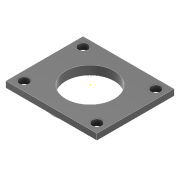
# Autodesk Inventor part: PinholeFlexFixture
Saved by Autodesk Inventor 2022 (Build 260153000, 153)
## iProperties
Created: 2022-02-18
Part Number: PinholeFlexFixture
Material: Acetal Resin, Black
Document SubType Name: Modeling
Designer: eganc
Density: 1.425 g/cm^3
Appearance: Smooth - Black
Author: eganc
Autodesk Inventor part; units mm, degrees
ref_plane "YZ Plane" through (0, 0, 0) normal (1, 0, 0) x (0, 1, 0)
ref_plane "XZ Plane" through (0, 0, 0) normal (0, 1, 0) x (-1, 0, 0)
ref_plane "XY Plane" through (0, 0, 0) normal (0, 0, 1) x (1, 0, 0)
sketch "Sketch1" plane through (0, 0, 0) normal (0, 1, 0) x (-1, 0, 0)
  line L0 (-7.5, 6.36) -> (7.5, 6.36)
  line L1 (7.5, 6.36) -> (7.5, -6.36)
  line L2 (7.5, -6.36) -> (-7.5, -6.36)
  line L3 (-7.5, -6.36) -> (-7.5, 6.36)
  line L4 (-7.5, 6.36) -> (7.5, -6.36) construction
  line L5 (7.5, 6.36) -> (-7.5, -6.36) construction
  point P0 (0, 0)
  dimension "d0" = 12.72
  dimension "d1" = 15
  constraints: 12 end point, 2 midpoint, 2 parallel, 1 horizontal, 1 perpendicular
  measures "d0" distance of L0.end L1.end
  measures "d1" distance of L1.end L2.end
extrude "Extrusion1" add sketch "Sketch1" along normal blind 1
sketch "Sketch2" plane through (0, 1, 0) normal (0, 1, 0) x (1, 0, 0)
  circle A0 centre (0, 0) radius 4
  dimension "d4" = 8
  constraints: 1 centre point, 1 coincident
  measures "d4" diameter of A0
extrude "Extrusion2" cut sketch "Sketch2" against normal up to surface (1 mm away)
sketch "Sketch3" plane through (0, 0, 0) normal (0, -1, 0) x (1, 0, 0)
  circle A0 centre (0, 0) radius 4
  circle A1 centre (0, 0) radius 6
  dimension "d7" = 12
  dimension "d8" = 8
  constraints: 2 centre point, 2 coincident
  measures "d7" diameter of A1
  measures "d8" diameter of A0
extrude "Extrusion3" add sketch "Sketch3" along normal blind 0.46
sketch "Sketch4" plane through (0, 1, 0) normal (0, 1, 0) x (1, 0, 0)
  point P0 (0, 0)
sketch "Sketch5" plane through (0, 1, 0) normal (0, 1, 0) x (1, 0, 0)
  circle A0 centre (-6, -4.86) radius 0.8
  line L0 (-7.5, 6.36) -> (-7.5, -6.36) projected
  line L1 (-7.5, 0) -> (7.5, 0) construction
  line L2 (7.5, -6.36) -> (7.5, 6.36) projected
  line L3 (-7.5, -6.36) -> (7.5, -6.36) projected
  line L4 (0, -6.36) -> (0, 6.36) construction
  line L5 (7.5, 6.36) -> (-7.5, 6.36) projected
  circle A1 centre (-6, 4.86) radius 0.8
  line L6 (0, 6.36) -> (0, -6.36) construction
  circle A2 centre (6, -4.86) radius 0.8
  circle A3 centre (6, 4.86) radius 0.8
  point P0 (0, 0)
  dimension "d11" = 1.5
  dimension "d12" = 1.6
  dimension "d13" = 1.5
  constraints: 6 end point, 5 symmetric about line, 4 centre point, 4 midpoint, 3 other
  measures "d11" distance from line of L3 A0.centre
  measures "d12" diameter of A0
  measures "d13" distance from line of L0 A0.centre
extrude "Extrusion4" cut sketch "Sketch5" against normal up to surface (1 mm away) contours A0 | A1 | A2 | A3
body "Solid1"
